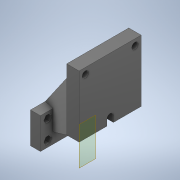
# Autodesk Inventor part: Soporte
Saved by Autodesk Inventor 2020.3 (Build 243373000, 373)
## iProperties
Created: 2020-11-02
Part Number: Soporte
Material: ABS Plastic
Document SubType Name: Modeling
Designer: juanp
Density: 1.06 g/cm^3
Appearance: Smooth - White
Author: juanp
Autodesk Inventor part; units mm, degrees
ref_plane "YZ Plane" through (0, 0, 0) normal (1, 0, 0) x (0, 1, 0)
ref_plane "XZ Plane" through (0, 0, 0) normal (0, 1, 0) x (-1, 0, 0)
ref_plane "XY Plane" through (0, 0, 0) normal (0, 0, 1) x (1, 0, 0)
sketch "Sketch1" plane through (0, 0, 0) normal (1, 0, 0) x (0, 1, 0)
  circle A0 centre (0, 0) radius 1.75
  circle A1 centre (15, 0) radius 1.75
  line L0 (15, 0) -> (0, 0) construction
  line L1 (15, 0) -> (15, 51.4) construction
  line L2 (0, 0) -> (0, 51.4) construction
  circle A2 centre (0, 51.4) radius 1.75
  circle A3 centre (15, 51.4) radius 1.75
  line L3 (15, 25.7) -> (15.4, 25.7) construction
  line L4 (20, 57.4) -> (-5, 57.4)
  line L5 (-5, 57.4) -> (-5, 45.4)
  line L6 (-5, 45.4) -> (20, 45.4)
  line L7 (20, 45.4) -> (20, 57.4)
  line L8 (20, 6) -> (-5, 6)
  line L9 (-5, 6) -> (-5, -6)
  line L10 (-5, -6) -> (20, -6)
  line L11 (20, -6) -> (20, 6)
  line L12 (7.5, 45.4) -> (7.5, 0) construction
  line L13 (15, 51.4) -> (20, 51.4) construction
  line L14 (15, 0) -> (20, 0)
  circle A4 centre (15.4, 25.7) radius 2.6
  line L15 (55.1, 45.7) -> (55.1, 5.7) construction
  circle A5 centre (55.1, 45.7) radius 2.6
  circle A6 centre (55.1, 5.7) radius 2.6
  line L16 (55.1, 25.7) -> (15.4, 25.7) construction
  dimension "d0" = 3.5
  dimension "d1" = 15
  dimension "d2" = 51.4
  dimension "d3" = 51.4
  dimension "d15" = 0.4
  dimension "d20" = 12
  dimension "d21" = 25
  dimension "d60" = 5.2
  dimension "d61" = 40
  dimension "d62" = 39.7
  constraints: 34 end point, 7 centre point, 7 horizontal, 6 coincident, 6 midpoint, 5 equal radius, 4 parallel, 3 perpendicular, 3 vertical, 2 collinear, 1 point on line
  measures "d0" diameter of A0
  measures "d1" distance of point (0, 0) L0.start
  measures "d2" distance of L0.start L1.end
  measures "d3" distance of L0.end L2.end
  measures "d15" distance of L3.end L3.start
  measures "d20" distance of L6.end L4.start
  measures "d21" distance of L9.end L10.end
  measures "d60" diameter of A4
  measures "d61" distance of L15.start L15.end
  measures "d62" distance of L16.start L16.end
extrude "Extrusion3" add sketch "Sketch1" along normal blind 8 contours L7 L6 L5 L4 | L11 L10 L9 L8
sketch "Sketch3" plane through (0, -5, -6) normal (0, -1, 0) x (1, 0, 0)
  arc A0 (0, 51.4) -> (0, 12) centre (-22.6254, 31.7) ccw construction
  arc A1 (8, 51.4) -> (8, 12) centre (-14.6254, 31.7) ccw construction
  line L0 (0, 51.4) -> (0, 63.4) projected
  line L1 (0, 63.4) -> (8, 63.4) projected
  line L2 (8, 51.4) -> (8, 63.4) projected
  line L3 (0, 51.4) -> (8, 51.4) projected
  line L4 (0, 0) -> (0, 12) projected
  line L5 (0, 12) -> (8, 12) projected
  line L6 (8, 0) -> (8, 12) projected
  line L7 (0, 0) -> (8, 0) projected
  arc A2 (8, 12) -> (8, 51.4) centre (-14.6254, 31.7) ccw
  arc A3 (0, 12) -> (0, 51.4) centre (-22.6254, 31.7) ccw
  point P0 (0, 6)
  dimension "d24" = 60
  constraints: 12 point on circle, 4 centre point, 4 end point, 1 equal radius
  measures "d24" diameter of A0
extrude "Extrusion4" add sketch "Sketch3" against normal up to surface (25 mm away) contours L3 A2 L5 A3
ref_plane "Work Plane1" through (32.5, 0, 0) normal (-1, 0, 0) x (0, 0, 1)
sketch "Sketch4" plane through (32.5, 0, 0) normal (-1, 0, 0) x (0, 0, 1)
  circle A0 centre (25.7, 15.4) radius 2.6 projected
  circle A1 centre (45.7, 55.1) radius 2.6 projected
  circle A2 centre (5.7, 55.1) radius 2.6 projected
  line L0 (25.7, 15) -> (25.7, 15.4) construction
  line L1 (50.7, 10.4) -> (0.7, 10.4)
  line L2 (0.7, 10.4) -> (0.7, 60.1)
  line L3 (0.7, 60.1) -> (50.7, 60.1)
  line L4 (50.7, 60.1) -> (50.7, 10.4)
  line L5 (28.3, 10.4) -> (28.3, 15.4)
  line L6 (23.1, 10.4) -> (23.1, 15.4)
  point P0 (25.7, 55.1)
  dimension "d67" = 5
  dimension "d68" = 5
  dimension "d69" = 5
  dimension "d70" = 5
  constraints: 12 end point, 3 parallel, 2 perpendicular, 2 point on circle, 2 point on line, 2 tangent, 1 horizontal
  measures "d67" distance from line of L1 A0.centre
  measures "d68" distance from line of L3 A1.centre
  measures "d69" distance from line of L4 A1.centre
  measures "d70" distance from line of L2 A2.centre
extrude "Extrusion5" add sketch "Sketch4" along normal blind 10 contours A0 L6 L1 L2 L3 L4 L5
sketch "Sketch8" plane through (8, 0, 0) normal (1, 0, 0) x (0, 0, -1)
  circle A0 centre (-51.4, 0) radius 1.75 projected
  line L0 (-54.6909, 0) -> (-53.0454, 2.85)
  line L1 (-53.0454, 2.85) -> (-49.7546, 2.85)
  line L2 (-49.7546, 2.85) -> (-48.1091, 0)
  line L3 (-48.1091, 0) -> (-49.7546, -2.85)
  line L4 (-49.7546, -2.85) -> (-53.0454, -2.85)
  line L5 (-53.0454, -2.85) -> (-54.6909, 0)
  circle A1 centre (-51.4, 15) radius 1.75 projected
  line L6 (-54.6909, 15) -> (-53.0454, 17.85)
  line L7 (-53.0454, 17.85) -> (-49.7546, 17.85)
  line L8 (-49.7546, 17.85) -> (-48.1091, 15)
  line L9 (-48.1091, 15) -> (-49.7546, 12.15)
  line L10 (-49.7546, 12.15) -> (-53.0454, 12.15)
  line L11 (-53.0454, 12.15) -> (-54.6909, 15)
  line L12 (-3.2909, 0) -> (-1.6454, 2.85)
  line L13 (-1.6454, 2.85) -> (1.6454, 2.85)
  line L14 (1.6454, 2.85) -> (3.2909, 0)
  line L15 (3.2909, 0) -> (1.6454, -2.85)
  line L16 (1.6454, -2.85) -> (-1.6454, -2.85)
  line L17 (-1.6454, -2.85) -> (-3.2909, 0)
  circle A2 centre (0, 15) radius 1.75 projected
  line L18 (-3.2909, 15) -> (-1.6454, 17.85)
  line L19 (-1.6454, 17.85) -> (1.6454, 17.85)
  line L20 (1.6454, 17.85) -> (3.2909, 15)
  line L21 (3.2909, 15) -> (1.6454, 12.15)
  line L22 (1.6454, 12.15) -> (-1.6454, 12.15)
  line L23 (-1.6454, 12.15) -> (-3.2909, 15)
  circle A3 centre (0, 0) radius 1.75 projected
  dimension "d54" = 5.7
  constraints: 48 end point, 4 coincident, 4 horizontal, 3 equal length, 52 other
  measures "d54" distance between parallel lines of L19 L22
extrude "Extrusion7" cut sketch "Sketch8" against normal blind 3.5 contours A0 | L0 L1 L2 L3 L4 L5 | A1 | L6 L7 L8 L9 L10 L11 | L12 L13 L14 L15 L16 L17 | A2 | L18 L19 L20 L21 L22 L23 | A3
sketch "Sketch10" plane through (22.5, 0, 0) normal (-1, 0, 0) x (0, 0, 1)
  line L0 (50.7, 10.4) -> (50.7, 60.1) projected
  line L1 (50.7, 50.1) -> (40.7, 50.1)
  line L2 (40.7, 50.1) -> (40.7, 35.25)
  line L3 (40.7, 10.4) -> (50.7, 10.4)
  line L4 (50.7, 10.4) -> (50.7, 50.1)
  line L5 (0.7, 10.4) -> (50.7, 10.4) projected
  line L6 (0.7, 60.1) -> (0.7, 10.4) projected
  line L7 (10.7, 10.4) -> (0.7, 10.4)
  line L8 (0.7, 10.4) -> (0.7, 50.1)
  line L9 (0.7, 50.1) -> (10.7, 50.1)
  line L10 (10.7, 50.1) -> (10.7, 35.25)
  line L11 (40.7, 30.25) -> (10.7, 30.25) construction
  line L12 (25.7, 35.25) -> (25.7, 25.25) construction
  line L13 (40.7, 35.25) -> (10.7, 35.25)
  line L14 (40.7, 25.25) -> (10.7, 25.25)
  line L15 (10.7, 30.25) -> (0.7, 30.25) construction
  circle A0 centre (5.7, 55.1) radius 2.6 projected
  line L16 (10.7, 25.25) -> (10.7, 10.4)
  line L17 (10.7, 35.25) -> (10.7, 25.25) construction
  line L18 (40.7, 35.25) -> (40.7, 25.25) construction
  line L19 (40.7, 25.25) -> (40.7, 10.4)
  point P0 (0, 0)
  point P1 (25.7, 30.25)
  dimension "d71" = 10
  dimension "d72" = 5
  constraints: 34 end point, 9 parallel, 6 midpoint, 5 horizontal, 5 point on line, 4 perpendicular, 2 collinear, 2 equal length, 1 vertical
  measures "d71" distance of L11.end L15.end
  measures "d72" distance from line of A0.centre L9
sketch "Sketch13" plane through (0, 0, 0) normal (-1, 0, 0) x (0, 0, 1)
  line L0 (45.4, 20) -> (57.4, 20) projected
  line L1 (57.4, -5) -> (45.4, -5) projected
  line L2 (6, -5) -> (45.4, -5) projected
  line L3 (35.4, 5) -> (16, 5)
  line L4 (-6, 20) -> (6, 20) projected
  line L5 (6, 20) -> (16, 20)
  line L6 (6, 20) -> (45.4, 20) projected
  line L7 (16, 20) -> (16, 15)
  line L8 (16, 15) -> (35.4, 15)
  line L9 (35.4, 15) -> (35.4, 20)
  line L10 (35.4, 20) -> (45.4, 20)
  line L11 (45.4, -5) -> (45.4, 20) projected
  line L12 (45.4, 20) -> (45.4, 0)
  line L13 (35.4, 5) -> (35.4, 0)
  line L14 (35.4, 0) -> (45.4, 0)
  line L15 (6, 20) -> (6, 0)
  line L16 (6, 20) -> (6, -5) projected
  line L17 (6, 0) -> (16, 0)
  line L18 (16, 0) -> (16, 5)
  point P0 (0, 0)
  dimension "d83" = 10
  dimension "d84" = 5
  dimension "d85" = 10
  constraints: 24 end point, 5 collinear, 4 perpendicular, 4 point on line, 2 horizontal, 1 vertical
  measures "d83" distance between parallel lines of L3 L8
  measures "d84" distance between parallel lines of L2 L14
  measures "d85" distance of L15.end L17.end
loft "Loft3" add profiles "Sketch10", "Sketch13" contours L3 L19 L14 L16 L5 L6 L9 L10 L13 L2 L1 L0 / L15 L5 L7 L8 L9 L6 L11 L14 L13 L3 L18 L17
sketch "Sketch14" plane through (0, -5, -6) normal (0, -1, 0) x (1, 0, 0)
  arc A0 (0, 12) -> (0, 51.4) centre (-22.6254, 31.7) ccw projected
  circle A1 centre (-22.6254, 31.7) radius 30
  point P0 (0, 6)
  point P1 (0, 51.4)
  point P2 (0, 12)
  constraints: 1 centre point, 1 coincident, 1 concentric
extrude "Extrusion10" cut sketch "Sketch14" against normal through all
sketch "Sketch15" plane through (32.5, 10.4, 0.7) normal (0, 0, -1) x (-1, 0, 0)
  line L0 (10, 0) -> (24.5, -6.7022) projected
  line L1 (24.5, -15.4) -> (24.5, -6.7022) projected
  line L2 (24.5, -6.7022) -> (24.5, -15.4)
  line L3 (24.5, -15.4) -> (10, -15.4)
  line L4 (10, 0) -> (10, 39.7) projected
  line L5 (10, -15.4) -> (10, 0)
  point P0 (32.5, -10.4)
  constraints: 6 end point, 2 perpendicular, 1 vertical
extrude "Extrusion11" cut sketch "Sketch15" against normal through all
body "Solid2"
